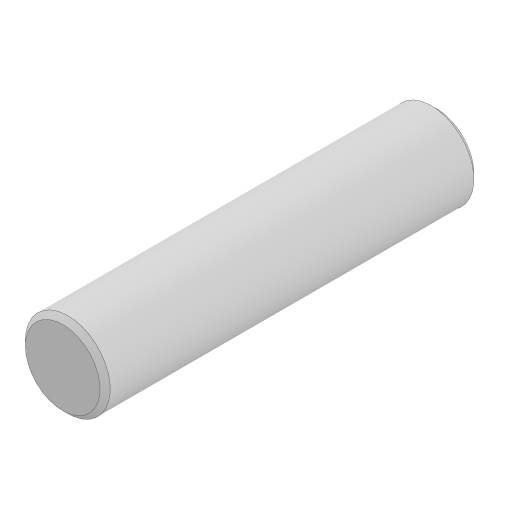
# Autodesk Inventor part: batt_10440
Saved by Autodesk Inventor 2023 (Build 270158000, 158)
## iProperties
Created: 2023-09-13
Part Number: batt_10440
Material: Generic
Document SubType Name: Modeling
Designer: James
Density: 1 g/cm^3
Appearance: Default
Author: James
Autodesk Inventor part; units mm, degrees
ref_plane "YZ Plane" through (0, 0, 0) normal (1, 0, 0) x (0, 1, 0)
ref_plane "XZ Plane" through (0, 0, 0) normal (0, 1, 0) x (-1, 0, 0)
ref_plane "XY Plane" through (0, 0, 0) normal (0, 0, 1) x (1, 0, 0)
sketch "Sketch2" plane through (0, 0, 0) normal (0, 1, 0) x (-1, 0, 0)
  line L0 (0, 0) -> (5, 0)
  line L1 (5, 0) -> (5, -44)
  line L2 (5, -44) -> (2, -44)
  line L3 (2, -44) -> (2, -45.5)
  line L4 (2, -45.5) -> (0, -45.5)
  line L5 (0, -45.5) -> (0, 0)
  line L6 (0, -54.6) -> (0, 9.1) projected
  dimension "d3" = 5
  dimension "d4" = 44
  dimension "d5" = 3
  dimension "d6" = 1.5
  constraints: 12 end point, 5 perpendicular, 1 horizontal
  measures "d3" distance of L0.start L0.end
  measures "d4" distance of L0.end L1.end
  measures "d5" distance of L1.end L2.end
  measures "d6" distance of L2.end L3.end
revolve "Revolution1" add sketch "Sketch2" angle 360 about axis through (0, 0, -10) along (0, 0, 1)
chamfer "Chamfer1" distance 0.6 angle 45 3 edges at (5, 0, 0) (5, 0, -44) (2, 0, -45.5)
body "Solid2"
